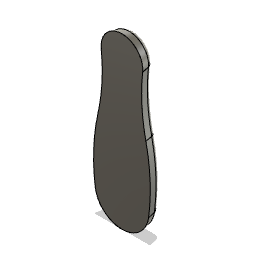
Link2 (Autodesk Fusion 360 design; units mm, degrees)
Autodesk Fusion 360 part; units mm, degrees
sketch "Sketch2" plane through (0, 0, 0) normal (0, 0, 1) x (1, 0, 0)
  arc A0 (29.8304, 196.8149) -> (35.2531, 100) centre (328.1348, 164.9639) ccw
  arc A1 (39.6352, -5.3902) -> (35.2531, 100) centre (-257.6286, 35.0361) ccw
  line L0 (0, 200) -> (0, 0) construction
  arc A2 (-35.2531, 100) -> (-29.8304, 196.8149) centre (-328.1348, 164.9639) ccw
  arc A3 (-35.2531, 100) -> (-39.6352, -5.3902) centre (257.6286, 35.0361) ccw
  arc A4 (29.8304, 196.8149) -> (-29.8304, 196.8149) centre (0, 200) ccw
  arc A5 (-39.6352, -5.3902) -> (39.6352, -5.3902) centre (0, 0) ccw
  dimension "d5" = 80
  dimension "d6" = 60
  dimension "d7" = 200
  dimension "d8" = 100
  dimension "d9" = 300
  constraint coincident L0.end A5.centre
  constraint vertical L0.end L0.start
  constraint tangent A0 A1
  constraint tangent A0 A4
  constraint tangent A1 A5
  constraint equal A0 A1
  constraint coincident L0.start A4.centre
  constraint symmetric A0.start L0 A2.end
  constraint symmetric A0.end L0 A2.start
  constraint symmetric A0 L0 A2
  constraint symmetric A1.start L0 A3.end
  constraint symmetric A1 L0 A3
  measures "d5" diameter of A5
  measures "d6" diameter of A4
  measures "d7" distance of L0.end L0.start
  measures "d8" vertical distance of L0.end A0.end
  measures "d9" radius of A0
extrude "Extrude1" add sketch "Sketch2" along normal blind 20
draft "Draft1" angle 12 neutral plane through (0, 0, 0) pull (0, 0, -1) 6 faces at (28.9556, 142.7876, 13.3333) (-25.9506, 215.0521, 13.3333) (-33.1008, 110.6047, 6.6667) (-37.5779, 88.451, 6.6667) (39.3319, -7.28, 13.3333) (40.9931, 6.3119, 13.3333)
fillet "Fillet1" radius 10 6 edges at (-28.6043, 148.1869, 0) (-42.1125, 47.499, 0) (0, -40, 0) (42.1125, 47.499, 0) (28.6043, 148.1869, 0) (0, 230, 0)
shell "Shell4" [suppressed]
ref_plane "WorkPlane1" through (0, 98.0755, 15) normal (0, 0, 1) x (1, 0, 0)
sketch "Sketch3" plane through (0, 98.0755, 15) normal (0, 0, 1) x (1, 0, 0)
  line L0 (-10, 90) -> (10, 90)
  line L1 (-10, 40) -> (10, 40)
  line L2 (-20, -20) -> (10, -20)
  line L3 (-20, -70) -> (20, -70)
  line L4 (-10, -113.3333) -> (9.4128, -113.3333)
  line L5 (-10, 20) -> (-10, -10)
  line L6 (10, 20) -> (10, -10)
  constraint horizontal L0
  constraint horizontal L1
  constraint horizontal L2
  constraint horizontal L3
  constraint horizontal L4
  constraint perpendicular L2 L5
  constraint vertical L6
web "Web1" [suppressed]
sketch "Sketch4" plane through (0, 0, 0) normal (0, 1, 0) x (1, 0, 0)
  line L0 (-9, -3) -> (9, -15)
rib "Rib1" [suppressed]
